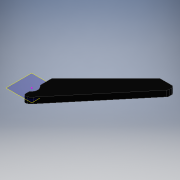
# Autodesk Inventor part: 頭_サブフレーム_1_1
Saved by Autodesk Inventor 2018 (Build 220112000, 112)
## iProperties
Created: 2016-06-01
Part Number: 頭_サブフレーム_1_1
Material: アセタール樹脂、黒
Document SubType Name: Modeling
Designer: hiroaki
Density: 1.425 g/cm^3
Appearance: 滑らか - 黒
Mass: 5.06992 g
Surface Area: 40.7842 cm^2
Volume: 3.55784 cm^3
Author: hiroaki
Autodesk Inventor part; units mm, degrees
ref_plane "YZ Plane" through (0, 0, 0) normal (1, 0, 0) x (0, 1, 0)
ref_plane "XZ Plane" through (0, 0, 0) normal (0, 1, 0) x (-1, 0, 0)
ref_plane "XY Plane" through (0, 0, 0) normal (0, 0, 1) x (1, 0, 0)
sketch "スケッチ1" plane through (0, 0, 0) normal (0, 0, 1) x (1, 0, 0)
  circle A0 centre (0, 0) radius 11 construction
  circle A1 centre (0, 8.5) radius 1.35
  circle A2 centre (0, 8.5) radius 2.5 construction
  circle A3 centre (0, 0) radius 5.05 construction
  circle A4 centre (0, -8.5) radius 1.35
  line L0 (48.7145, 60.75) -> (2.55, 14.5855)
  line L1 (0, 0) -> (0, 48.2635) construction
  line L2 (60.75, 60.75) -> (0, 0) construction
  line L3 (48.7145, 60.75) -> (60.75, 60.75)
  line L4 (60.75, 60.75) -> (60.75, 55.75)
  arc A5 (2.55, -10.7004) -> (8.4522, -7.0399) centre (0, 0) ccw
  line L5 (60.75, 55.75) -> (8.4522, -7.0399)
  circle A6 centre (0, 0) radius 8.5 construction
  circle A7 centre (8.5, 0) radius 1.35
  line L6 (2.55, 14.5855) -> (2.55, 4.3589)
  arc A8 (2.55, -4.3589) -> (2.55, 4.3589) centre (0, 0) ccw
  line L7 (2.55, -4.3589) -> (2.55, -10.7004)
  dimension "d3" = 10.1
  dimension "d0" = 2.7
  dimension "d1" = 8.5
  dimension "d2" = 5
  dimension "d6" = 360
  dimension "d11" = 45
  dimension "d13" = 60.75
  dimension "d17" = 5
  dimension "d18" = 2.55
  constraints: 16 end point, 8 centre point, 6 coincident, 6 point on circle, 3 tangent, 3 vertical, 2 vertical alignment, 1 concentric, 1 equal radius, 1 horizontal, 1 horizontal alignment, 1 parallel, 1 perpendicular, 10 other
  measures "d0" diameter of A1
  measures "d1" distance of A1.centre point (0, 0)
  measures "d2" diameter of A2
  measures "d11" angle of L1 L2
  measures "d13" horizontal distance of L2.start point (0, 0)
  measures "d17" distance of L2.start L4.end
  measures "d18" distance from line of L6 A1.centre
extrude "押し出し1" add sketch "スケッチ1" along normal blind 5 contours L3 L4 L5 A5 L7 A8 L6 L0
fillet "フィレット1" radius 2 7 edges at (2.55, -10.7004, 2.5) (2.55, -4.3589, 2.5) (2.55, 14.5855, 2.5) (60.75, 60.75, 2.5) (60.75, 55.75, 2.5) (48.7145, 60.75, 2.5) (2.55, 4.3589, 2.5)
sketch "スケッチ3" plane through (0, 0, 0) normal (0, 0, -1) x (-1, 0, 0)
  circle A0 centre (-8.5, 0) radius 1.35 projected
  circle A1 centre (-8.5, 0) radius 1.35
  point P0 (0, 0)
  constraints: 1 centre point, 1 coincident
extrude "押し出し3" add sketch "スケッチ3" against normal up to surface (5 mm away) from surface at 0
ref_plane "作業平面1" through (0, 0, 4) normal (0, 0, -1) x (-1, 0, 0)
sketch "スケッチ4" plane through (0, 0, 4) normal (0, 0, -1) x (-1, 0, 0)
  point P0 (0, 0)
